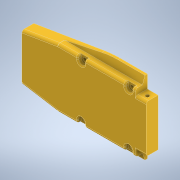
# Autodesk Inventor part: BodyStructure Side
Saved by Autodesk Inventor 2022.2 (Build 262287000, 287)
## iProperties
Created: 2022-01-14
Part Number: BodyStructure Side
Material: Generic
Document SubType Name: Modeling
Designer: Jochen
Density: 1 g/cm^3
Appearance: Default
Author: Jochen
Autodesk Inventor part; units mm, degrees
ref_plane "YZ Plane" through (0, 0, 0) normal (1, 0, 0) x (0, 1, 0)
ref_plane "XZ Plane" through (0, 0, 0) normal (0, 1, 0) x (-1, 0, 0)
ref_plane "Work Plane1" through (0, 0, 50) normal (0, 0, 1) x (1, 0, 0)
sketch "Sketch1" plane through (0, 0, 50) normal (0, 0, 1) x (1, 0, 0)
  line L0 (0, -20) -> (0, 20)
  line L1 (0, 20) -> (-9, 20)
  line L2 (-9, -31) -> (-32, -31)
  line L3 (-45.0709, -29.925) -> (-105, -20)
  line L4 (-105, -20) -> (-105, 20)
  line L5 (-105, 20) -> (-45.0709, 29.925)
  line L6 (-32, 31) -> (-9, 31)
  line L7 (-9, 31) -> (-9, 20)
  line L8 (-9, -20) -> (0, -20)
  line L9 (0, -68.6) -> (0, 68.6) construction
  line L10 (-126, 0) -> (21, 0) construction
  line L11 (-9, -20) -> (-9, -31)
  arc A0 (-45.0709, -29.925) -> (-32, -31) centre (-32, 49) ccw
  arc A1 (-32, 31) -> (-45.0709, 29.925) centre (-32, -49) ccw
  point P0 (0, 0)
  dimension "d2" = 105
  dimension "d3" = 40
  dimension "d4" = 9
  dimension "d6" = 80
  dimension "d7" = 40
  dimension "d8" = 62
  dimension "d9" = 23
  constraints: 20 end point, 4 perpendicular, 4 point on circle, 4 tangent, 2 centre point, 2 parallel, 1 equal radius, 1 point on line, 1 vertical, 4 other
  measures "d2" distance between parallel lines of L4 L9
  measures "d3" distance of L0.start L0.end
  measures "d4" distance between parallel lines of L9 L11
  measures "d6" radius of A0
  measures "d7" distance of L3.end L4.end
  measures "d8" distance between parallel lines of L6 L2
  measures "d9" distance of L2.start L2.end
extrude "Extrusion1" add sketch "Sketch1" along normal blind 10
sketch "Sketch2" plane through (0, 0, 50) normal (0, 0, 1) x (1, 0, 0)
  circle A0 centre (-55, -22) radius 1.5
  circle A1 centre (-15, -22) radius 1.5
  circle A2 centre (-55, 22) radius 1.5
  circle A3 centre (-15, 22) radius 1.5
  line L0 (-4, -10) -> (-4, 10) construction
  line L1 (-5.5, -10) -> (-5.5, 10)
  line L2 (-2.5, 10) -> (-2.5, -10)
  arc A4 (-5.5, -10) -> (-2.5, -10) centre (-4, -10) ccw
  arc A5 (-2.5, 10) -> (-5.5, 10) centre (-4, 10) ccw
  line L3 (-105, -11) -> (-97, -11)
  line L4 (-95, -9) -> (-95, 9)
  line L5 (-97, 11) -> (-105, 11)
  line L6 (-105, 11) -> (-105, -11)
  arc A6 (-97, -11) -> (-95, -9) centre (-97, -9) ccw
  arc A7 (-95, 9) -> (-97, 11) centre (-97, 9) ccw
  line L7 (0, -20) -> (-9, -20) projected
  line L8 (-9, -20) -> (-9, -31) projected
  line L9 (-9, -31) -> (-32, -31) projected
  arc A8 (-45.0709, -29.925) -> (-32, -31) centre (-32, 49) ccw projected
  line L10 (-45.0709, -29.925) -> (-105, -20) projected
  line L11 (-105, -20) -> (-105, 20) projected
  line L12 (-105, 20) -> (-45.0709, 29.925) projected
  arc A9 (-32, 31) -> (-45.0709, 29.925) centre (-32, -49) ccw projected
  line L13 (-32, 31) -> (-9, 31) projected
  line L14 (-9, 31) -> (-9, 20) projected
  line L15 (-9, 20) -> (0, 20) projected
  line L16 (0, 20) -> (0, -20) projected
  line L17 (0, -20) -> (-9, -20) projected
  line L18 (-9, -20) -> (-9, -31) projected
  line L19 (-9, -31) -> (-32, -31) projected
  arc A10 (-45.0709, -29.925) -> (-32, -31) centre (-32, 49) ccw projected
  line L20 (-45.0709, -29.925) -> (-105, -20) projected
  line L21 (-105, -20) -> (-105, 20) projected
  line L22 (-105, 20) -> (-45.0709, 29.925) projected
  arc A11 (-32, 31) -> (-45.0709, 29.925) centre (-32, -49) ccw projected
  line L23 (-32, 31) -> (-9, 31) projected
  line L24 (-9, 31) -> (-9, 20) projected
  line L25 (-9, 20) -> (0, 20) projected
  line L26 (0, 20) -> (0, -20) projected
  line L27 (0, -68.6) -> (0, 68.6) construction
  line L28 (-126, 0) -> (21, 0) construction
  line L29 (-105, 20) -> (-105, -20) construction
  arc A12 (-52, -22) -> (-58, -22) centre (-55, -22) ccw
  arc A13 (-12, -22) -> (-18, -22) centre (-15, -22) ccw
  arc A14 (-58, 22) -> (-52, 22) centre (-55, 22) ccw
  arc A15 (-18, 22) -> (-12, 22) centre (-15, 22) ccw
  line L30 (-7, -15) -> (-7, 15)
  arc A16 (-7, 15) -> (-9, 17) centre (-9, 15) ccw
  line L31 (-9, 17) -> (-15, 17)
  arc A17 (-19.7916, 20.5714) -> (-15, 17) centre (-15, 22) ccw
  line L32 (-21.7082, 22) -> (-47.8121, 22)
  arc A18 (-52.8042, 17) -> (-54, 15.1688) centre (-52, 15.1688) ccw
  line L33 (-54, 15.1688) -> (-54, -15.1688)
  arc A19 (-54, -15.1688) -> (-52.8042, -17) centre (-52, -15.1688) ccw
  line L34 (-47.8121, -22) -> (-21.7082, -22)
  arc A20 (-15, -17) -> (-19.7916, -20.5714) centre (-15, -22) ccw
  line L35 (-15, -17) -> (-9, -17)
  arc A21 (-9, -17) -> (-7, -15) centre (-9, -15) ccw
  arc A22 (-52.8042, 17) -> (-49.7389, 20.5361) centre (-55, 22) ccw
  arc A23 (-19.7916, 20.5714) -> (-21.7082, 22) centre (-21.7082, 20) ccw
  arc A24 (-47.8121, 22) -> (-49.7389, 20.5361) centre (-47.8121, 20) ccw
  line L36 (-55, -22) -> (-55, 22) construction
  line L37 (-56, -15.1688) -> (-56, 15.1688)
  arc A25 (-49.7389, -20.5361) -> (-52.8042, -17) centre (-55, -22) ccw
  arc A26 (-49.7389, -20.5361) -> (-47.8121, -22) centre (-47.8121, -20) ccw
  arc A27 (-21.7082, -22) -> (-19.7916, -20.5714) centre (-21.7082, -20) ccw
  arc A28 (-56, 15.1688) -> (-57.1958, 17) centre (-58, 15.1688) ccw
  arc A29 (-60.2611, 20.5361) -> (-57.1958, 17) centre (-55, 22) ccw
  arc A30 (-60.2611, 20.5361) -> (-62.1879, 22) centre (-62.1879, 20) ccw
  line L38 (-62.1879, 22) -> (-74.3977, 22)
  arc A31 (-74.3977, 22) -> (-74.7245, 21.9731) centre (-74.3977, 20) ccw
  line L39 (-74.7245, 21.9731) -> (-91.3268, 19.2236)
  arc A32 (-91.3268, 19.2236) -> (-93, 17.2505) centre (-91, 17.2505) ccw
  line L40 (-93, 17.2505) -> (-93, -17.2505)
  arc A33 (-93, -17.2505) -> (-91.3268, -19.2236) centre (-91, -17.2505) ccw
  line L41 (-91.3268, -19.2236) -> (-74.7245, -21.9731)
  arc A34 (-57.1958, -17) -> (-56, -15.1688) centre (-58, -15.1688) ccw
  arc A35 (-57.1958, -17) -> (-60.2611, -20.5361) centre (-55, -22) ccw
  arc A36 (-74.7245, -21.9731) -> (-74.3977, -22) centre (-74.3977, -20) ccw
  line L42 (-74.3977, -22) -> (-62.1879, -22)
  arc A37 (-62.1879, -22) -> (-60.2611, -20.5361) centre (-62.1879, -20) ccw
  line L43 (-58, -22) -> (-58, -27.7838)
  line L44 (-52, -22) -> (-52, -28.7774)
  line L45 (-105, -20) -> (-45.0709, -29.925) projected
  line L46 (-18, -22) -> (-18, -31)
  line L47 (-12, -22) -> (-12, -31)
  line L48 (-12, 22) -> (-12, 31)
  line L49 (-9, 31) -> (-32, 31) projected
  line L50 (-18, 22) -> (-18, 31)
  line L51 (-52, 22) -> (-52, 28.7774)
  line L52 (-58, 22) -> (-58, 27.7838)
  line L53 (-45.0709, 29.925) -> (-105, 20) projected
  point P0 (0, 0)
  point P1 (-4, 0)
  point P2 (-105, 0)
  dimension "d12" = 2
  dimension "d13" = 22
  dimension "d14" = 10
  dimension "d15" = 3
  dimension "d16" = 6
  dimension "d17" = 44
  dimension "d18" = 44
  dimension "d20" = 55
  dimension "d21" = 15
  dimension "d22" = 4
  dimension "d23" = 20
  dimension "d24" = 1.5
  dimension "d25" = 3
  dimension "d26" = 2
  dimension "d27" = 2
  dimension "d28" = 44
  dimension "d29" = 2
  dimension "d30" = 2
  dimension "d31" = 3
  constraints: 61 point on circle, 58 end point, 43 tangent, 34 centre point, 18 point on line, 14 equal radius, 7 parallel, 7 vertical, 4 coincident, 3 midpoint, 3 perpendicular, 2 concentric, 2 symmetric about line, 1 collinear, 1 horizontal, 19 other
  measures "d12" radius of A6
  measures "d13" distance of L5.end L3.start
  measures "d14" distance between parallel lines of L11 L4
  measures "d15" diameter of A1
  measures "d16" diameter of A13
  measures "d17" distance of A2.centre A0.centre
  measures "d18" distance of A3.centre A1.centre
  measures "d20" distance from line of L16 A0.centre
  measures "d21" distance from line of L27 A1.centre
  measures "d22" distance between parallel lines of L27 L0
  measures "d23" distance of L0.start L0.end
  measures "d24" radius of A4
  measures "d25" distance between parallel lines of L0 L30
  measures "d26" radius of A16
  measures "d27" radial gap between concentric circles of A15 A17
  measures "d28" distance between parallel lines of L32 L34
  measures "d29" distance between parallel lines of L33 L37
  measures "d30" distance between parallel lines of L40 L4
  measures "d31" distance between parallel lines of L10 L41
extrude "Extrusion2" cut sketch "Sketch2" along normal blind 9 contours L1 A5 L2 A4 | L6 L5 A7 L4 A6 L3 | A21 L35 A20 A27 L34 A26 A25 A19 L33 A18 A22 A24 L32 A23 A17 L31 A16 L30 | A34 A35 A37 L42 A36 L41 A33 L40 A32 L39 A31 L38 A30 A29 A28 L37
sketch "Sketch3" plane through (0, 0, 0) normal (1, 0, 0) x (0, 1, 0)
  line L0 (0, -18.0828) -> (0, 73.4971) construction
  line L1 (-43.4, 0) -> (43.4, 0) construction
  line L2 (-31, 50.0602) -> (-20, 50.0602) construction
  line L3 (-20, 50) -> (-20, 60) construction
  line L4 (-31.0006, 50) -> (-30.9976, 60) construction
  line L5 (20, 50) -> (31, 50) construction
  line L6 (-31, 50) -> (-31, 52)
  line L7 (-25, 54.1838) -> (-25, 58)
  line L8 (-31, 52) -> (-25, 54.1838)
  line L9 (-23, 60) -> (23, 60)
  line L10 (25, 58) -> (25, 54.1838)
  line L11 (29.925, 50) -> (20, 50) projected
  line L12 (25, 54.1838) -> (31, 52)
  line L13 (31, 50) -> (-31, 50)
  line L14 (31, 52) -> (31, 50)
  line L15 (20, 60) -> (20, 50) construction
  line L16 (20, 50) -> (-20, 50) construction
  line L17 (-20, 50) -> (-20, 60) construction
  line L18 (-20, 60) -> (20, 60) construction
  line L19 (20, 60) -> (20, 50) construction
  line L20 (20, 50) -> (-20, 50) construction
  line L21 (-20, 50) -> (-20, 60) construction
  line L22 (-20, 60) -> (20, 60) construction
  line L23 (20, 50) -> (31, 50) construction
  line L24 (31, 50) -> (31, 60) construction
  line L25 (20, 60) -> (31, 60) construction
  line L26 (20, 50) -> (20, 60) construction
  line L27 (-20, 50) -> (20, 50) construction
  line L28 (20, 50) -> (20, 60) construction
  line L29 (-20, 60) -> (20, 60) construction
  line L30 (-20, 50) -> (-20, 60) construction
  line L31 (-31, 50) -> (-20, 50) construction
  line L32 (-20, 50) -> (-20, 60) construction
  line L33 (-31, 60) -> (-20, 60) construction
  line L34 (-31, 50) -> (-31, 60) construction
  arc A0 (-23, 60) -> (-25, 58) centre (-23, 58) ccw
  arc A1 (25, 58) -> (23, 60) centre (23, 58) ccw
  point P0 (0, 0)
  point P1 (25, 56.0919)
  dimension "d35" = 20
  dimension "d36" = 50
  dimension "d37" = 2
  dimension "d38" = 46
  constraints: 18 end point, 4 point on circle, 4 point on line, 4 tangent, 2 centre point, 1 coincident, 1 midpoint, 1 parallel, 1 perpendicular, 1 vertical, 5 other
  measures "d35" angle of L2 L8
  measures "d36" distance from line of point (25, 56.092) L7
  measures "d37" distance of L2.start L6.end
  measures "d38" distance of L9.end L9.start
extrude "Extrusion4" cut sketch "Sketch3" against normal through all keep common part
extrude "Extrusion5" cut sketch "Sketch2" against normal blind 3 from surface at 10 contours A0 | A1 | A2 | A3 | L43 A12 L44 L10 | L12 L51 A14 L52 | L46 A13 L47 L9 | L13 L48 A15 L50
extrude "Extrusion6" cut sketch "Sketch2" along normal through all contours A0 | A1 | A2 | A3
fillet "Fillet1" radius 1 28 edges at (-18, 24.4142, 59.4142) (-18, 25, 57.5) (-15, 19, 60) (-12, 22.5, 60) (-12, 24.4142, 59.4142) (-12, 25, 57.5) (-18, 22.5, 60) (-58, 25, 57.5) (-58, 22.5, 60) (-55, 19, 60) (-52, 22.5, 60) (-52, 24.4142, 59.4142) (-52, 25, 57.5) (-58, 24.4142, 59.4142) (-52, -22.5, 60) (-52, -24.4142, 59.4142) (-52, -25, 57.5) (-58, -22.5, 60) (-58, -24.4142, 59.4142) (-58, -25, 57.5) (-55, -19, 60) (-12, -22.5, 60) (-12, -24.4142, 59.4142) (-12, -25, 57.5) (-18, -22.5, 60) (-18, -24.4142, 59.4142) (-18, -25, 57.5) (-15, -19, 60)
fillet "Fillet1" radius 2 2 edges at (-4.5, 20, 60) (-4.5, -20, 60)
fillet "Fillet1" radius 2 6 edges at (-78.346, -24.4142, 59.4142) (-74.8089, -25, 56.0919) (-95.9427, -21.5, 60) (-78.346, 24.4142, 59.4142) (-74.8089, 25, 56.0919) (-95.9427, 21.5, 60)
sketch "Sketch4" plane through (0, 0, 0) normal (0, 1, 0) x (-1, 0, 0)
  line L0 (0, -11.8) -> (0, 70.8) construction
  line L1 (10.8, 0) -> (-1.8, 0) construction
  circle A0 centre (4, 55) radius 1.5
  line L2 (5.5, 50) -> (5.5, 59) construction
  line L3 (9, 50) -> (0, 50) construction
  point P0 (0, 0)
  dimension "d52" = 3
  dimension "d53" = 5
  constraints: 1 centre point, 1 tangent
  measures "d52" diameter of A0
  measures "d53" distance from line of L3 A0.centre
extrude "Extrusion7" cut sketch "Sketch4" along normal through all both and the other way through all
sketch "Sketch5" plane through (0, 0, 0) normal (1, 0, 0) x (0, 1, 0)
  circle A0 centre (15, 55) radius 1.5
  circle A1 centre (-15, 55) radius 1.5
  line L0 (-10, 50) -> (10, 50) projected
  line L1 (0, -11.3) -> (0, 67.8) construction
  line L2 (-23.1, 0) -> (23.1, 0) construction
  point P0 (0, 0)
  dimension "d56" = 3
  dimension "d57" = 5
  dimension "d58" = 30
  constraints: 2 centre point, 1 equal radius, 1 symmetric about line
  measures "d56" diameter of A1
  measures "d57" distance from line of L0 A1.centre
  measures "d58" distance of A0.centre A1.centre
extrude "Extrusion8" cut sketch "Sketch5" along normal blind 10 from surface at -105
equation "\"d18\" = d17"
body "Solid1"
